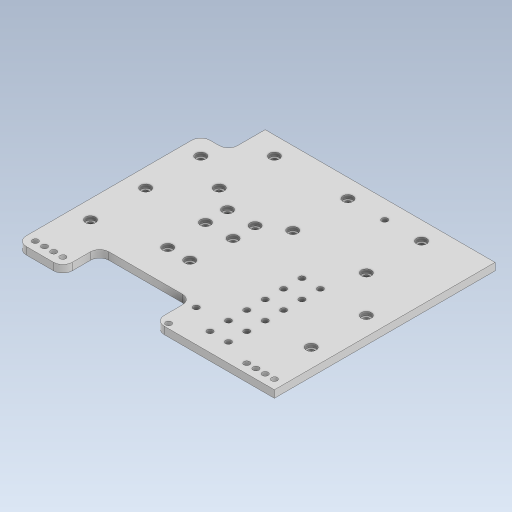
# Autodesk Inventor part: Fix Casis Kiri Bawah
Saved by Autodesk Inventor 2023.5 (Build 275446000, 446)
## iProperties
Created: 2025-10-01
Part Number: Fix Casis Kiri Bawah
Material: Generic
Document SubType Name: Modeling
Designer: Guntur
Density: 1 g/cm^3
Appearance: Default
Author: Guntur
## iProperties of the stored document Fix Casis Kiri Depan_3DPrint.ipt
Created: 2025-10-17
Part Number: Fix Casis Kiri Depan_3DPrint
Material: Generic
Document SubType Name: Modeling
Designer: Guntur
Density: 1 g/cm^3
Appearance: Default
Author: Guntur
Autodesk Inventor part; units mm, degrees
ref_plane "YZ Plane" through (0, 0, 0) normal (1, 0, 0) x (0, 1, 0)
ref_plane "XZ Plane" through (0, 0, 0) normal (0, 1, 0) x (-1, 0, 0)
ref_plane "XY Plane" through (0, 0, 0) normal (0, 0, 1) x (1, 0, 0)
sketch "Sketch1" plane through (0, 0, 0) normal (0, 1, 0) x (-1, 0, 0)
  line L0 (0, 0) -> (-140, 0)
  line L1 (-140, 0) -> (-140, -120)
  line L2 (-140, -120) -> (0, -120)
  line L3 (0, -120) -> (0, 0)
  line L4 (-25, 0) -> (-75, 0)
  line L5 (-75, 0) -> (-75, -20)
  line L6 (-75, -20) -> (-25, -20)
  line L7 (-25, -20) -> (-25, 0)
  circle A0 centre (-5, -5) radius 1.6
  circle A1 centre (-10, -5) radius 1.6
  circle A2 centre (-15, -5) radius 1.6
  circle A3 centre (-20, -5) radius 1.6
  circle A4 centre (-130, -30) radius 1.6
  line L8 (0, -60) -> (-140, -60) construction
  line L9 (-70, -120) -> (-70, 0) construction
  circle A5 centre (-135, -5) radius 1.6
  circle A6 centre (-130, -5) radius 1.6
  circle A7 centre (-125, -5) radius 1.6
  circle A8 centre (-120, -5) radius 1.6
  circle A9 centre (-130, -60) radius 1.6
  circle A10 centre (-130, -30) radius 2.75
  circle A11 centre (-130, -60) radius 2.75
  circle A12 centre (-5, -115) radius 1.6
  circle A13 centre (-10, -115) radius 1.6
  circle A14 centre (-30, -110) radius 1.6
  circle A15 centre (-30, -110) radius 2.75
  circle A16 centre (-110, -110) radius 1.6
  circle A17 centre (-110, -110) radius 2.75
  circle A18 centre (-70, -110) radius 1.6
  circle A19 centre (-70, -110) radius 2.75
  circle A20 centre (-44, -38) radius 1.6
  circle A21 centre (-44, -38) radius 2.75
  circle A22 centre (-56, -38) radius 1.6
  circle A23 centre (-56, -38) radius 2.75
  circle A24 centre (-57.5, -60) radius 1.6
  circle A25 centre (-57.5, -60) radius 2.75
  circle A26 centre (-57.5, -72) radius 1.6
  circle A27 centre (-57.5, -72) radius 2.75
  circle A28 centre (-42.5, -60) radius 1.6
  circle A29 centre (-42.5, -60) radius 2.75
  circle A30 centre (-42.5, -72) radius 1.6
  circle A31 centre (-42.5, -72) radius 2.75
  circle A32 centre (-10, -30) radius 1.6
  circle A33 centre (-10, -60) radius 1.6
  circle A34 centre (-10, -30) radius 2.75
  circle A35 centre (-10, -60) radius 2.75
  circle A36 centre (-10, -90) radius 1.6
  circle A37 centre (-10, -90) radius 2.75
  circle A38 centre (-80, -2.5) radius 1.6
  circle A39 centre (-80, -17.5) radius 1.6
  circle A40 centre (-105, -10) radius 1.6
  circle A41 centre (-105, -20) radius 1.6
  circle A42 centre (-95, -20) radius 1.6
  circle A43 centre (-95, -10) radius 1.6
  circle A44 centre (-95, -30) radius 1.6
  circle A45 centre (-95, -40) radius 1.6
  circle A46 centre (-105, -30) radius 1.6
  circle A47 centre (-105, -40) radius 1.6
  circle A48 centre (-95, -50) radius 1.6
  circle A49 centre (-95, -60) radius 1.6
  circle A50 centre (-105, -50) radius 1.6
  circle A51 centre (-105, -60) radius 1.6
  circle A52 centre (-110, -80) radius 1.65
  circle A53 centre (-110, -80) radius 2.75
  circle A54 centre (-70, -80) radius 1.65
  circle A55 centre (-70, -80) radius 2.75
  circle A56 centre (-30, -80) radius 1.65
  circle A57 centre (-30, -80) radius 2.75
  line L10 (0, -120) -> (-15, -120)
  line L11 (-15, -120) -> (-15, -100)
  line L12 (-15, -100) -> (0, -100)
  line L13 (0, -100) -> (0, -120)
  circle A58 centre (-90, -110) radius 1.6
  point P0 (-50, -38)
  point P1 (-50, -74.6125)
  dimension "d0" = 140
  dimension "d1" = 120
  dimension "d2" = 50
  dimension "d3" = 20
  dimension "d4" = 25
  dimension "d5" = 3.2
  dimension "d6" = 5
  dimension "d7" = 5
  dimension "d8" = 3.2
  dimension "d9" = 5
  dimension "d10" = 3.2
  dimension "d11" = 5
  dimension "d12" = 3.2
  dimension "d13" = 5
  dimension "d14" = 3.2
  dimension "d15" = 10
  dimension "d16" = 30
  dimension "d17" = 3.2
  dimension "d18" = 5.5
  dimension "d19" = 5.5
  dimension "d20" = 3.2
  dimension "d22" = 5.5
  dimension "d23" = 3.2
  dimension "d24" = 5.5
  dimension "d28" = 3.2
  dimension "d30" = 5.5
  dimension "d34" = 3.2
  dimension "d37" = 5.5
  dimension "d42" = 30
  dimension "d43" = 10
  dimension "d44" = 10
  dimension "d46" = 10
  dimension "d47" = 3.2
  dimension "d48" = 5
  dimension "d49" = 2.5
  dimension "d50" = 3.2
  dimension "d51" = 15
  dimension "d52" = 3.2
  dimension "d53" = 3.2
  dimension "d54" = 10
  dimension "d55" = 3.2
  dimension "d56" = 10
  dimension "d57" = 3.2
  dimension "d58" = 20
  dimension "d59" = 10
  dimension "d60" = 10
  dimension "d61" = 3.2
  dimension "d62" = 10
  dimension "d63" = 3.2
  dimension "d64" = 10
  dimension "d65" = 3.2
  dimension "d66" = 3.2
  dimension "d67" = 3.2
  dimension "d68" = 10
  dimension "d69" = 3.2
  dimension "d70" = 10
  dimension "d71" = 3.2
  dimension "d72" = 3.2
  dimension "d73" = 3.3
  dimension "d74" = 5.5
  dimension "d76" = 3.3
  dimension "d77" = 5.5
  dimension "d78" = 30
  dimension "d79" = 30
  constraints: 59 centre point, 28 end point, 17 coincident, 14 symmetric about line, 6 parallel, 6 point on line, 4 perpendicular, 3 horizontal, 3 midpoint, 14 other
  measures "d0" distance of L2.end L1.end
  measures "d1" distance of L1.end L0.end
  measures "d2" distance of L6.end L5.end
  measures "d3" distance of L5.end L4.end
  measures "d4" distance between parallel lines of L3 L7
  measures "d5" diameter of A0
  measures "d6" distance from line of L3 A0.centre
  measures "d7" distance from line of L0 A0.centre
  measures "d8" diameter of A1
  measures "d9" distance of A1.centre A0.centre
  measures "d10" diameter of A2
  measures "d11" distance of A2.centre A1.centre
  measures "d12" diameter of A3
  measures "d13" distance of A3.centre A2.centre
  measures "d14" diameter of A4
  measures "d15" distance from line of L1 A4.centre
  measures "d16" distance from line of L0 A4.centre
  measures "d17" diameter of A9
  measures "d18" diameter of A10
  measures "d19" diameter of A11
  measures "d20" diameter of A14
  measures "d22" diameter of A15
  measures "d23" diameter of A18
  measures "d24" diameter of A19
  measures "d28" diameter of A20
  measures "d30" diameter of A21
  measures "d34" diameter of A24
  measures "d37" diameter of A25
  measures "d42" distance from line of A14.centre L3
  measures "d43" distance from line of L2 A14.centre
  measures "d44" distance from line of L2 A18.centre
  measures "d46" distance of L8.end A9.centre
  measures "d47" diameter of A38
  measures "d48" distance from line of L5 A38.centre
  measures "d49" distance from line of L0 A38.centre
  measures "d50" diameter of A39
  measures "d51" distance of A39.centre A38.centre
  measures "d52" diameter of A40
  measures "d53" diameter of A41
  measures "d54" distance of A41.centre A40.centre
  measures "d55" diameter of A42
  measures "d56" distance of A41.centre A42.centre
  measures "d57" diameter of A43
  measures "d58" distance from line of L5 A43.centre
  measures "d59" distance of A40.centre A43.centre
  measures "d60" distance from line of L0 A43.centre
  measures "d61" diameter of A44
  measures "d62" distance of A44.centre A42.centre
  measures "d63" diameter of A45
  measures "d64" distance of A45.centre A44.centre
  measures "d65" diameter of A46
  measures "d66" diameter of A47
  measures "d67" diameter of A48
  measures "d68" distance of A48.centre A45.centre
  measures "d69" diameter of A49
  measures "d70" distance of A49.centre A48.centre
  measures "d71" diameter of A50
  measures "d72" diameter of A51
  measures "d73" diameter of A52
  measures "d74" diameter of A53
  measures "d76" diameter of A54
  measures "d77" diameter of A55
  measures "d78" distance of A17.centre A52.centre
  measures "d79" distance of A18.centre A54.centre
extrude "Extrusion1" add sketch "Sketch1" along normal blind 4 contours L3 L12 L11 L2 L1 L0 L5 L6 L7
extrude "Extrusion2" add sketch "Sketch1" along normal blind 2 contours A10 | A11 | A15 | A17 | A19 | A21 | A23 | A25 | A27 | A29 | A31 | A34 | A35 | A37 | A53 | A55 | A57
fillet "Fillet1" radius 5 7 edges at (15, 2, -100) (0, 2, -100) (75, 2, 0) (25, 2, 0) (0, 2, 0) (75, 2, -20) (25, 2, -20)
body "Solid1"
